Autodesk Fusion 360 part; units mm, degrees
note: some values were not read from the file. Set by a fixed rule: which sketch regions a step uses.
(part 11 of 15)
  line L8809 (248.7, -65.336) -> (248.925, -65.5074)
  line L8810 (248.339, -68.8671) -> (248.069, -68.9523)
  line L8811 (-57.7847, -68.2576) -> (-57.7166, -67.9835)
  line L8812 (-50.3027, -70.2857) -> (-50.4682, -70.3693)
  line L8813 (-55.7831, -66.6017) -> (-55.5017, -66.6261)
  line L8814 (249.602, -67.0076) -> (249.598, -67.1332)
  line L8815 (-57.536, -69.6196) -> (-57.6623, -69.3669)
  line L8816 (248.925, -65.5074) -> (249.123, -65.7087)
  line L8817 (-50.4436, -68.6079) -> (-50.2805, -68.696)
  line L8818 (-51.192, -70.3542) -> (-51.3539, -70.2637)
  line L8819 (249.598, -67.1332) -> (249.561, -67.4132)
  line L8820 (248.069, -68.9523) -> (247.791, -68.9987)
  line L8821 (-49.8621, -69.5102) -> (-49.8853, -69.6941)
  line L8822 (-55.0783, -70.4611) -> (-55.3476, -70.5462)
  line L8823 (249.291, -65.9359) -> (249.425, -66.1846)
  line L8824 (249.582, -66.7258) -> (249.602, -67.0076)
  line L8825 (-53.8561, -69.0071) -> (-53.9328, -69.279)
  line L8826 (-51.7461, -69.6551) -> (-51.7616, -69.4704)
  line L8827 (-51.4951, -70.1436) -> (-51.6102, -69.9983)
  line L8828 (-50.0204, -68.9579) -> (-49.9334, -69.1216)
  line L8829 (-51.6849, -69.1094) -> (-51.5956, -68.9469)
  line L8830 (-50.6467, -70.4192) -> (-50.8316, -70.4334)
  line L8831 (-51.1676, -68.6028) -> (-50.9897, -68.5505)
  line L8832 (-51.0157, -70.4115) -> (-51.192, -70.3542)
  line L8833 (-56.1893, -70.5661) -> (-56.4624, -70.4937)
  line L8834 (-51.7409, -69.2861) -> (-51.6849, -69.1094)
  line L8835 (-51.695, -69.8334) -> (-51.7461, -69.6551)
  line L8836 (-51.3319, -68.6887) -> (-51.1676, -68.6028)
  line L8837 (246.452, -68.6439) -> (246.233, -68.4655)
  line L8838 (246.233, -68.4655) -> (246.041, -68.2581)
  line L8839 (-51.6102, -69.9983) -> (-51.695, -69.8334)
  line L8840 (-49.8798, -69.2991) -> (-49.8617, -69.4836)
  line L8841 (249.484, -67.6851) -> (249.37, -67.9434)
  line L8842 (-50.0354, -70.0312) -> (-50.1566, -70.1716)
  line L8843 (248.828, -68.5879) -> (248.593, -68.7448)
  line L8844 (249.123, -65.7087) -> (249.291, -65.9359)
  line L8845 (-50.2805, -68.696) -> (-50.1376, -68.8142)
  line L8846 (-54.047, -69.5374) -> (-54.1965, -69.7771)
  line L8847 (-50.1566, -70.1716) -> (-50.3027, -70.2857)
  line L8848 (-49.9438, -69.87) -> (-50.0354, -70.0312)
  line L8849 (-51.3539, -70.2637) -> (-51.4951, -70.1436)
  line L8850 (-49.9334, -69.1216) -> (-49.8798, -69.2991)
  line L8851 (-51.7616, -69.4704) -> (-51.7409, -69.2861)
  line L8852 (-51.5956, -68.9469) -> (-51.4764, -68.8049)
  line L8853 (-50.9897, -68.5505) -> (-50.8051, -68.5337)
  line L8854 (249.039, -68.3994) -> (248.828, -68.5879)
  line L8855 (-50.6207, -68.553) -> (-50.4436, -68.6079)
  line L8856 (-50.4682, -70.3693) -> (-50.6467, -70.4192)
  line L8857 (-53.9328, -69.279) -> (-54.047, -69.5374)
  line L8858 (-57.8024, -68.821) -> (-57.8135, -68.5387)
  line L8859 (-49.8617, -69.4836) -> (-49.8621, -69.5102)
  line L8860 (-57.3754, -69.852) -> (-57.536, -69.6196)
  line L8861 (-57.8135, -68.5387) -> (-57.7847, -68.2576)
  line L8862 (-57.7517, -69.0989) -> (-57.8024, -68.821)
  line L8863 (-55.9087, -70.5993) -> (-56.1893, -70.5661)
  line L8864 (-57.4687, -67.4773) -> (-57.2938, -67.2555)
  line L8865 (-54.3783, -69.9933) -> (-54.5887, -70.1818)
  line L8866 (-50.8316, -70.4334) -> (-51.0157, -70.4115)
  line L8867 (-51.4764, -68.8049) -> (-51.3319, -68.6887)
  line L8868 (-50.1376, -68.8142) -> (-50.0204, -68.9579)
  line L8869 (-55.6263, -70.5926) -> (-55.9087, -70.5993)
  line L8870 (-56.0652, -66.6173) -> (-55.7831, -66.6017)
  line L8871 (-49.8853, -69.6941) -> (-49.9438, -69.87)
  line L8872 (88.5197, -67.9034) -> (88.3702, -68.1431)
  line L8873 (88.7322, -66.6857) -> (88.7522, -66.9675)
  line L8874 (246.328, -65.4666) -> (246.557, -65.3023)
  line L8875 (245.7, -66.3896) -> (245.806, -66.1277)
  line L8876 (247.634, -65.0078) -> (247.915, -65.0322)
  line L8877 (245.614, -67.2271) -> (245.603, -66.9448)
  line L8878 (86.3774, -68.9321) -> (86.1043, -68.8597)
  line L8879 (84.7819, -66.6237) -> (84.85, -66.3495)
  line L8880 (85.9579, -65.132) -> (86.2244, -65.0384)
  line L8881 (248.593, -68.7448) -> (248.339, -68.8671)
  line L8882 (245.603, -66.9448) -> (245.632, -66.6637)
  line L8883 (85.4773, -65.4265) -> (85.7072, -65.2622)
  line L8884 (243.131, -67.1021) -> (243.274, -67.2203)
  line L8885 (249.425, -66.1846) -> (249.523, -66.4496)
  line L8886 (86.6579, -68.9653) -> (86.3774, -68.9321)
  line L8887 (85.3831, -68.4255) -> (85.1913, -68.218)
  line L8888 (87.3402, -65.0559) -> (87.6037, -65.1579)
  line L8889 (87.8502, -65.2959) -> (88.0748, -65.4673)
  line L8890 (-50.8051, -68.5337) -> (-50.6207, -68.553)
  line L8891 (246.955, -68.8998) -> (246.694, -68.7896)
  line L8892 (87.065, -64.9921) -> (87.3402, -65.0559)
  line L8893 (245.806, -66.1277) -> (245.948, -65.8834)
  line L8894 (247.791, -68.9987) -> (247.508, -69.0054)
  line L8895 (88.7482, -67.0931) -> (88.7106, -67.3731)
  line L8896 (248.19, -65.096) -> (248.454, -65.1979)
  line L8897 (88.4408, -65.8959) -> (88.575, -66.1445)
  line L8898 (88.7522, -66.9675) -> (88.7482, -67.0931)
  line L8899 (247.352, -65.0234) -> (247.634, -65.0078)
  line L8900 (87.6037, -65.1579) -> (87.8502, -65.2959)
  line L8901 (88.273, -65.6686) -> (88.4408, -65.8959)
  line L8902 (88.3702, -68.1431) -> (88.1884, -68.3593)
  line L8903 (246.041, -68.2581) -> (245.881, -68.0257)
  line L8904 (247.915, -65.0322) -> (248.19, -65.096)
  line L8905 (245.632, -66.6637) -> (245.7, -66.3896)
  line L8906 (248.454, -65.1979) -> (248.7, -65.336)
  line L8907 (84.7531, -66.9047) -> (84.7819, -66.6237)
  line L8908 (84.85, -66.3495) -> (84.9561, -66.0876)
  line L8909 (88.6727, -66.4095) -> (88.7322, -66.6857)
  line L8910 (86.2244, -65.0384) -> (86.5015, -64.9833)
  line L8911 (246.808, -65.1721) -> (247.075, -65.0785)
  line L8912 (249.523, -66.4496) -> (249.582, -66.7258)
  line L8913 (88.7106, -67.3731) -> (88.6339, -67.645)
  line L8914 (88.0748, -65.4673) -> (88.273, -65.6686)
  line L8915 (247.228, -68.9722) -> (246.955, -68.8998)
  line L8916 (249.22, -68.1832) -> (249.039, -68.3994)
  line L8917 (245.665, -67.505) -> (245.614, -67.2271)
  line L8918 (246.557, -65.3023) -> (246.808, -65.1721)
  line L8919 (249.561, -67.4132) -> (249.484, -67.6851)
  line L8920 (246.694, -68.7896) -> (246.452, -68.6439)
  line L8921 (88.1884, -68.3593) -> (87.978, -68.5478)
  line L8922 (88.575, -66.1445) -> (88.6727, -66.4095)
  line L8923 (86.9404, -68.9586) -> (86.6579, -68.9653)
  line L8924 (245.755, -67.773) -> (245.665, -67.505)
  line L8925 (84.9044, -67.7329) -> (84.815, -67.4649)
  line L8926 (86.7836, -64.9678) -> (87.065, -64.9921)
  line L8927 (242.791, -66.9591) -> (242.968, -67.0139)
  line L8928 (246.123, -65.6616) -> (246.328, -65.4666)
  line L8929 (85.8442, -68.7495) -> (85.6021, -68.6038)
  line L8930 (85.1913, -68.218) -> (85.0307, -67.9856)
  line L8931 (247.075, -65.0785) -> (247.352, -65.0234)
  line L8932 (247.508, -69.0054) -> (247.228, -68.9722)
  line L8933 (245.881, -68.0257) -> (245.755, -67.773)
  line L8934 (88.6339, -67.645) -> (88.5197, -67.9034)
  line L8935 (245.948, -65.8834) -> (246.123, -65.6616)
  line L8936 (243.549, -67.9162) -> (243.526, -68.1002)
  line L8937 (241.816, -67.353) -> (241.935, -67.211)
  line L8938 (243.255, -68.5777) -> (243.109, -68.6918)
  line L8939 (241.67, -67.6922) -> (241.726, -67.5155)
  line L8940 (86.1043, -68.8597) -> (85.8442, -68.7495)
  line L8941 (242.58, -68.8395) -> (242.396, -68.8176)
  line L8942 (87.978, -68.5478) -> (87.7431, -68.7048)
  line L8943 (84.815, -67.4649) -> (84.7642, -67.187)
  line L8944 (243.109, -68.6918) -> (242.943, -68.7754)
  line L8945 (241.665, -68.0612) -> (241.65, -67.8765)
  line L8946 (243.467, -68.2761) -> (243.376, -68.4373)
  line L8947 (87.7431, -68.7048) -> (87.4884, -68.8271)
  line L8948 (242.943, -68.7754) -> (242.764, -68.8253)
  line L8949 (242.422, -66.9565) -> (242.606, -66.9397)
  line L8950 (85.0307, -67.9856) -> (84.9044, -67.7329)
  line L8951 (91.946, -66.9191) -> (92.1231, -66.9739)
  line L8952 (243.526, -68.1002) -> (243.467, -68.2761)
  line L8953 (85.098, -65.8434) -> (85.2729, -65.6215)
  line L8954 (243.478, -67.5277) -> (243.531, -67.7052)
  line L8955 (86.5015, -64.9833) -> (86.7836, -64.9678)
  line L8956 (242.396, -68.8176) -> (242.219, -68.7603)
  line L8957 (242.057, -68.6698) -> (241.916, -68.5496)
  line L8958 (241.716, -68.2394) -> (241.665, -68.0612)
  line L8959 (242.079, -67.0948) -> (242.244, -67.0089)
  line L8960 (91.2348, -67.0547) -> (91.3991, -66.9688)
  line L8961 (243.274, -67.2203) -> (243.391, -67.364)
  line L8962 (-60.4492, -66.8436) -> (-60.2861, -66.9318)
  line L8963 (92.6869, -67.6651) -> (92.705, -67.8497)
  line L8964 (92.6814, -68.0601) -> (92.6228, -68.2361)
  line L8965 (243.376, -68.4373) -> (243.255, -68.5777)
  line L8966 (92.264, -68.6518) -> (92.0985, -68.7354)
  line L8967 (92.705, -67.8497) -> (92.7046, -67.8762)
  line L8968 (91.7351, -68.7994) -> (91.551, -68.7775)
  line L8969 (92.0985, -68.7354) -> (91.9199, -68.7852)
  line L8970 (90.8206, -68.0211) -> (90.8051, -67.8364)
  line L8971 (92.7046, -67.8762) -> (92.6814, -68.0601)
  line L8972 (243.55, -67.8897) -> (243.549, -67.9162)
  line L8973 (241.65, -67.8765) -> (241.67, -67.6922)
  line L8974 (91.577, -66.9165) -> (91.7616, -66.8997)
  line L8975 (242.764, -68.8253) -> (242.58, -68.8395)
  line L8976 (242.606, -66.9397) -> (242.791, -66.9591)
  line L8977 (92.4101, -68.5376) -> (92.264, -68.6518)
  line L8978 (242.244, -67.0089) -> (242.422, -66.9565)
  line L8979 (241.726, -67.5155) -> (241.816, -67.353)
  line L8980 (91.2128, -68.6297) -> (91.0716, -68.5096)
  line L8981 (91.0716, -68.5096) -> (90.9564, -68.3643)
  line L8982 (85.2729, -65.6215) -> (85.4773, -65.4265)
  line L8983 (243.391, -67.364) -> (243.478, -67.5277)
  line L8984 (87.4884, -68.8271) -> (87.219, -68.9123)
  line L8985 (241.916, -68.5496) -> (241.801, -68.4043)
  line L8986 (243.531, -67.7052) -> (243.55, -67.8897)
  line L8987 (91.551, -68.7775) -> (91.3746, -68.7202)
  line L8988 (241.801, -68.4043) -> (241.716, -68.2394)
  line L8989 (84.7642, -67.187) -> (84.7531, -66.9047)
  line L8990 (241.935, -67.211) -> (242.079, -67.0948)
  line L8991 (92.2862, -67.0621) -> (92.4291, -67.1803)
  line L8992 (90.8717, -68.1994) -> (90.8206, -68.0211)
  line L8993 (242.219, -68.7603) -> (242.057, -68.6698)
  line L8994 (92.1231, -66.9739) -> (92.2862, -67.0621)
  line L8995 (87.219, -68.9123) -> (86.9404, -68.9586)
  line L8996 (85.6021, -68.6038) -> (85.3831, -68.4255)
  line L8997 (242.968, -67.0139) -> (243.131, -67.1021)
  line L8998 (84.9561, -66.0876) -> (85.098, -65.8434)
  line L8999 (85.7072, -65.2622) -> (85.9579, -65.132)
  line L9000 (-60.0261, -67.1936) -> (-59.939, -67.3574)
  line L9001 (-60.1433, -67.05) -> (-60.0261, -67.1936)
  line L9002 (-59.891, -67.9298) -> (-59.9495, -68.1058)
  line L9003 (-61.1732, -66.8385) -> (-60.9954, -66.7862)
  line L9004 (-60.6524, -68.6549) -> (-60.8372, -68.6692)
  line L9005 (-59.939, -67.3574) -> (-59.8854, -67.5348)
  line L9006 (-60.8372, -68.6692) -> (-61.0213, -68.6472)
  line L9007 (-60.1622, -68.4073) -> (-60.3083, -68.5215)
  line L9008 (-61.3595, -68.4995) -> (-61.5007, -68.3793)
  line L9009 (-60.8107, -66.7694) -> (-60.6263, -66.7888)
  line L9010 (-61.7673, -67.7061) -> (-61.7466, -67.5219)
  line L9011 (176.49, -67.4428) -> (176.44, -67.6091)
  line L9012 (90.9711, -67.3129) -> (91.0903, -67.1709)
  line L9013 (-61.0213, -68.6472) -> (-61.1977, -68.5899)
  line L9014 (-61.1977, -68.5899) -> (-61.3595, -68.4995)
  line L9015 (175.752, -66.56) -> (175.845, -66.5658)
  line L9016 (174.659, -68.0542) -> (174.491, -68.013)
  line L9017 (-60.2861, -66.9318) -> (-60.1433, -67.05)
  line L9018 (176.501, -67.2694) -> (176.49, -67.4428)
  line L9019 (92.5463, -67.3239) -> (92.6333, -67.4876)
  line L9020 (-60.9954, -66.7862) -> (-60.8107, -66.7694)
  line L9021 (-61.7466, -67.5219) -> (-61.6905, -67.3451)
  line L9022 (174.003, -67.3506) -> (174.014, -67.1772)
  line L9023 (91.9199, -68.7852) -> (91.7351, -68.7994)
  line L9024 (-61.6012, -67.1827) -> (-61.482, -67.0406)
  line L9025 (-59.9495, -68.1058) -> (-60.0411, -68.267)
  line L9026 (-61.3375, -66.9244) -> (-61.1732, -66.8385)
  line L9027 (176.471, -67.0982) -> (176.501, -67.2694)
  line L9028 (176.233, -67.8854) -> (176.088, -67.9806)
  line L9029 (-60.6263, -66.7888) -> (-60.4492, -66.8436)
  line L9030 (-61.5007, -68.3793) -> (-61.6159, -68.234)
  line L9031 (90.8051, -67.8364) -> (90.8257, -67.6521)
  line L9032 (-60.3083, -68.5215) -> (-60.4738, -68.6051)
  line L9033 (90.8818, -67.4754) -> (90.9711, -67.3129)
  line L9034 (-61.6159, -68.234) -> (-61.7006, -68.0691)
  line L9035 (174.151, -66.8607) -> (174.271, -66.7346)
  line L9036 (176.088, -67.9806) -> (175.925, -68.0399)
  line L9037 (175.845, -66.5658) -> (176.013, -66.607)
  line L9038 (92.5313, -68.3973) -> (92.4101, -68.5376)
  line L9039 (91.3991, -66.9688) -> (91.577, -66.9165)
  line L9040 (-61.6905, -67.3451) -> (-61.6012, -67.1827)
  line L9041 (-60.4738, -68.6051) -> (-60.6524, -68.6549)
  line L9042 (-59.8677, -67.7459) -> (-59.891, -67.9298)
  line L9043 (159.928, -66.686) -> (160.061, -66.7985)
  line L9044 (174.491, -68.013) -> (174.336, -67.934)
  line L9045 (174.579, -66.5801) -> (174.752, -66.56)
  line L9046 (174.014, -67.1772) -> (174.064, -67.0109)
  line L9047 (174.271, -66.7346) -> (174.416, -66.6394)
  line L9048 (176.168, -66.686) -> (176.301, -66.7985)
  line L9049 (-59.8854, -67.5348) -> (-59.8673, -67.7194)
  line L9050 (-61.7517, -67.8909) -> (-61.7673, -67.7061)
  line L9051 (174.101, -67.6816) -> (174.033, -67.5218)
  line L9052 (91.7616, -66.8997) -> (91.946, -66.9191)
  line L9053 (90.9564, -68.3643) -> (90.8717, -68.1994)
  line L9054 (92.4291, -67.1803) -> (92.5463, -67.3239)
  line L9055 (90.8257, -67.6521) -> (90.8818, -67.4754)
  line L9056 (91.0903, -67.1709) -> (91.2348, -67.0547)
  line L9057 (92.6228, -68.2361) -> (92.5313, -68.3973)
  line L9058 (-61.482, -67.0406) -> (-61.3375, -66.9244)
  line L9059 (-61.7006, -68.0691) -> (-61.7517, -67.8909)
  line L9060 (92.6333, -67.4876) -> (92.6869, -67.6651)
  line L9061 (-60.0411, -68.267) -> (-60.1622, -68.4073)
  line L9062 (91.3746, -68.7202) -> (91.2128, -68.6297)
  line L9063 (-59.8673, -67.7194) -> (-59.8677, -67.7459)
  line L9064 (158.339, -66.5801) -> (158.512, -66.56)
  line L9065 (268.083, -64.4506) -> (268.281, -64.652)
  line L9066 (159.512, -68.06) -> (158.512, -68.06)
  line L9067 (160.061, -66.7985) -> (160.163, -66.9384)
  line L9068 (267.611, -64.1412) -> (267.858, -64.2792)
  line L9069 (174.064, -67.0109) -> (174.151, -66.8607)
  line L9070 (268.76, -65.9509) -> (268.756, -66.0764)
  line L9071 (268.583, -65.1278) -> (268.68, -65.3929)
  line L9072 (268.281, -64.652) -> (268.449, -64.8792)
  line L9073 (268.68, -65.3929) -> (268.74, -65.6691)
  line L9074 (267.348, -64.0393) -> (267.611, -64.1412)
  line L9075 (264.772, -66.1703) -> (264.761, -65.888)
  line L9076 (264.858, -65.3328) -> (264.964, -65.071)
  line L9077 (176.013, -66.607) -> (176.168, -66.686)
  line L9078 (267.751, -67.6881) -> (267.496, -67.8104)
  line L9079 (264.964, -65.071) -> (265.106, -64.8267)
  line L9080 (159.993, -67.8854) -> (159.848, -67.9806)
  line L9081 (157.911, -66.8607) -> (158.031, -66.7346)
  line L9082 (174.752, -68.06) -> (174.659, -68.0542)
  line L9083 (176.403, -66.9384) -> (176.471, -67.0982)
  line L9084 (267.073, -63.9755) -> (267.348, -64.0393)
  line L9085 (160.261, -67.2694) -> (160.25, -67.4428)
  line L9086 (174.416, -66.6394) -> (174.579, -66.5801)
  line L9087 (159.685, -68.0399) -> (159.512, -68.06)
  line L9088 (174.752, -66.56) -> (175.752, -66.56)
  line L9089 (267.858, -64.2792) -> (268.083, -64.4506)
  line L9090 (160.231, -67.0982) -> (160.261, -67.2694)
  line L9091 (158.419, -68.0542) -> (158.251, -68.013)
  line L9092 (160.25, -67.4428) -> (160.2, -67.6091)
  line L9093 (160.113, -67.7593) -> (159.993, -67.8854)
  line L9094 (158.031, -66.7346) -> (158.176, -66.6394)
  line L9095 (176.353, -67.7593) -> (176.233, -67.8854)
  line L9096 (174.033, -67.5218) -> (174.003, -67.3506)
  line L9097 (158.176, -66.6394) -> (158.339, -66.5801)
  line L9098 (174.203, -67.8215) -> (174.101, -67.6816)
  line L9099 (267.227, -67.8956) -> (266.948, -67.942)
  line L9100 (266.112, -67.843) -> (265.852, -67.7329)
  line L9101 (157.861, -67.6816) -> (157.793, -67.5218)
  line L9102 (266.948, -67.942) -> (266.666, -67.9486)
  line L9103 (157.793, -67.5218) -> (157.763, -67.3506)
  line L9104 (159.605, -66.5658) -> (159.773, -66.607)
  line L9105 (158.512, -66.56) -> (159.512, -66.56)
  line L9106 (159.512, -66.56) -> (159.605, -66.5658)
  line L9107 (176.301, -66.7985) -> (176.403, -66.9384)
  line L9108 (159.773, -66.607) -> (159.928, -66.686)
  line L9109 (158.251, -68.013) -> (158.096, -67.934)
  line L9110 (157.774, -67.1772) -> (157.824, -67.0109)
  line L9111 (176.44, -67.6091) -> (176.353, -67.7593)
  line L9112 (174.336, -67.934) -> (174.203, -67.8215)
  line L9113 (160.163, -66.9384) -> (160.231, -67.0982)
  line L9114 (157.963, -67.8215) -> (157.861, -67.6816)
  line L9115 (268.378, -67.1264) -> (268.196, -67.3427)
  line L9116 (159.848, -67.9806) -> (159.685, -68.0399)
  line L9117 (268.642, -66.6283) -> (268.527, -66.8867)
  line L9118 (265.852, -67.7329) -> (265.61, -67.5872)
  line L9119 (265.61, -67.5872) -> (265.391, -67.4088)
  line L9120 (160.2, -67.6091) -> (160.113, -67.7593)
  line L9121 (158.512, -68.06) -> (158.419, -68.0542)
  line L9122 (268.718, -66.3564) -> (268.642, -66.6283)
  line L9123 (157.824, -67.0109) -> (157.911, -66.8607)
  line L9124 (175.925, -68.0399) -> (175.752, -68.06)
  line L9125 (175.752, -68.06) -> (174.752, -68.06)
  line L9126 (157.763, -67.3506) -> (157.774, -67.1772)
  line L9127 (158.096, -67.934) -> (157.963, -67.8215)
  line L9128 (67.7828, -67.9019) -> (67.5004, -67.9086)
  line L9129 (69.1154, -64.6119) -> (69.2833, -64.8391)
  line L9130 (67.2198, -67.8754) -> (66.9468, -67.803)
  line L9131 (261.948, -65.9024) -> (262.125, -65.9572)
  line L9132 (264.823, -66.4482) -> (264.772, -66.1703)
  line L9133 (266.791, -63.9511) -> (267.073, -63.9755)
  line L9134 (69.4174, -65.0878) -> (69.5152, -65.3528)
  line L9135 (267.986, -67.5312) -> (267.751, -67.6881)
  line L9136 (66.6866, -67.6928) -> (66.4446, -67.5471)
  line L9137 (266.666, -67.9486) -> (266.385, -67.9154)
  line L9138 (266.509, -63.9666) -> (266.791, -63.9511)
  line L9139 (265.966, -64.1153) -> (266.232, -64.0217)
  line L9140 (262.125, -65.9572) -> (262.288, -66.0454)
  line L9141 (67.0669, -63.9817) -> (67.3439, -63.9266)
  line L9142 (265.281, -64.6048) -> (265.485, -64.4098)
  line L9143 (262.288, -66.0454) -> (262.431, -66.1636)
  line L9144 (66.4446, -67.5471) -> (66.2255, -67.3687)
  line L9145 (69.5946, -65.9108) -> (69.5907, -66.0364)
  line L9146 (68.9172, -64.4106) -> (69.1154, -64.6119)
  line L9147 (69.0309, -67.3026) -> (68.8204, -67.4911)
  line L9148 (68.4462, -64.1011) -> (68.6927, -64.2392)
  line L9149 (69.5907, -66.0364) -> (69.5531, -66.3164)
  line L9150 (68.0615, -67.8555) -> (67.7828, -67.9019)
  line L9151 (69.5152, -65.3528) -> (69.5747, -65.629)
  line L9152 (69.4764, -66.5883) -> (69.3621, -66.8467)
  line L9153 (264.912, -66.7162) -> (264.823, -66.4482)
  line L9154 (68.8204, -67.4911) -> (68.5855, -67.6481)
  line L9155 (265.485, -64.4098) -> (265.715, -64.2456)
  line L9156 (268.756, -66.0764) -> (268.718, -66.3564)
  line L9157 (268.449, -64.8792) -> (268.583, -65.1278)
  line L9158 (69.2126, -67.0864) -> (69.0309, -67.3026)
  line L9159 (65.7986, -65.0309) -> (65.9404, -64.7866)
  line L9160 (65.6244, -65.5669) -> (65.6925, -65.2928)
  line L9161 (65.8731, -66.9289) -> (65.7468, -66.6762)
  line L9162 (262.707, -66.8595) -> (262.683, -67.0435)
  line L9163 (262.683, -67.0435) -> (262.625, -67.2194)
  line L9164 (265.715, -64.2456) -> (265.966, -64.1153)
  line L9165 (264.761, -65.888) -> (264.79, -65.607)
  line L9166 (265.199, -67.2013) -> (265.038, -66.9689)
  line L9167 (264.79, -65.607) -> (264.858, -65.3328)
  line L9168 (265.391, -67.4088) -> (265.199, -67.2013)
  line L9169 (68.3309, -67.7703) -> (68.0615, -67.8555)
  line L9170 (69.5531, -66.3164) -> (69.4764, -66.5883)
  line L9171 (66.0337, -67.1613) -> (65.8731, -66.9289)
  line L9172 (267.496, -67.8104) -> (267.227, -67.8956)
  line L9173 (268.74, -65.6691) -> (268.76, -65.9509)
  line L9174 (268.527, -66.8867) -> (268.378, -67.1264)
  line L9175 (268.196, -67.3427) -> (267.986, -67.5312)
  line L9176 (69.5747, -65.629) -> (69.5946, -65.9108)
  line L9177 (68.5855, -67.6481) -> (68.3309, -67.7703)
  line L9178 (265.106, -64.8267) -> (265.281, -64.6048)
  line L9179 (67.5004, -67.9086) -> (67.2198, -67.8754)
  line L9180 (68.1827, -63.9992) -> (68.4462, -64.1011)
  line L9181 (68.6927, -64.2392) -> (68.9172, -64.4106)
  line L9182 (65.5956, -65.848) -> (65.6244, -65.5669)
  line L9183 (67.9075, -63.9354) -> (68.1827, -63.9992)
  line L9184 (66.3198, -64.3698) -> (66.5496, -64.2055)
  line L9185 (65.6574, -66.4082) -> (65.6067, -66.1303)
  line L9186 (265.038, -66.9689) -> (264.912, -66.7162)
  line L9187 (69.2833, -64.8391) -> (69.4174, -65.0878)
  line L9188 (66.8003, -64.0753) -> (67.0669, -63.9817)
  line L9189 (266.232, -64.0217) -> (266.509, -63.9666)
  line L9190 (69.3621, -66.8467) -> (69.2126, -67.0864)
  line L9191 (266.385, -67.9154) -> (266.112, -67.843)
  line L9192 (72.941, -67.6786) -> (72.7624, -67.7285)
  line L9193 (71.7243, -66.4187) -> (71.8136, -66.2562)
  line L9194 (72.9656, -65.9172) -> (73.1287, -66.0053)
  line L9195 (261.377, -67.7035) -> (261.215, -67.6131)
  line L9196 (262.707, -66.833) -> (262.707, -66.8595)
  line L9197 (73.3887, -66.2672) -> (73.4758, -66.4309)
  line L9198 (262.635, -66.471) -> (262.689, -66.6485)
  line L9199 (261.764, -65.883) -> (261.948, -65.9024)
  line L9200 (261.092, -66.1542) -> (261.237, -66.0381)
  line L9201 (71.7989, -67.3075) -> (71.7141, -67.1426)
  line L9202 (286.857, -63.5848) -> (287.104, -63.7228)
  line L9203 (73.5293, -66.6084) -> (73.5474, -66.7929)
  line L9204 (287.104, -63.7228) -> (287.328, -63.8942)
  line L9205 (287.526, -64.0955) -> (287.694, -64.3228)
  line L9206 (262.548, -66.3073) -> (262.635, -66.471)
  line L9207 (261.579, -65.8998) -> (261.764, -65.883)
  line L9208 (72.2171, -67.6635) -> (72.0553, -67.573)
  line L9209 (65.6067, -66.1303) -> (65.5956, -65.848)
  line L9210 (262.689, -66.6485) -> (262.707, -66.833)
  line L9211 (67.626, -63.911) -> (67.9075, -63.9354)
  line L9212 (73.5474, -66.7929) -> (73.5471, -66.8195)
  line L9213 (262.412, -67.521) -> (262.266, -67.6351)
  line L9214 (73.5238, -67.0034) -> (73.4653, -67.1793)
  line L9215 (65.7468, -66.6762) -> (65.6574, -66.4082)
  line L9216 (260.884, -66.4587) -> (260.973, -66.2963)
  line L9217 (261.074, -67.4929) -> (260.959, -67.3476)
  line L9218 (260.828, -66.6355) -> (260.884, -66.4587)
  line L9219 (287.328, -63.8942) -> (287.526, -64.0955)
  line L9220 (260.973, -66.2963) -> (261.092, -66.1542)
  line L9221 (71.9141, -67.4528) -> (71.7989, -67.3075)
  line L9222 (66.5496, -64.2055) -> (66.8003, -64.0753)
  line L9223 (261.737, -67.7828) -> (261.553, -67.7608)
  line L9224 (260.959, -67.3476) -> (260.874, -67.1827)
  line L9225 (261.237, -66.0381) -> (261.401, -65.9522)
  line L9226 (72.0772, -65.998) -> (72.2416, -65.9121)
  line L9227 (287.694, -64.3228) -> (287.828, -64.5714)
  line L9228 (262.431, -66.1636) -> (262.548, -66.3073)
  line L9229 (286.319, -63.419) -> (286.594, -63.4828)
  line L9230 (262.533, -67.3806) -> (262.412, -67.521)
  line L9231 (73.3737, -67.3405) -> (73.2526, -67.4809)
  line L9232 (71.7141, -67.1426) -> (71.663, -66.9644)
  line L9233 (260.823, -67.0045) -> (260.807, -66.8197)
  line L9234 (262.625, -67.2194) -> (262.533, -67.3806)
  line L9235 (67.3439, -63.9266) -> (67.626, -63.911)
  line L9236 (65.9404, -64.7866) -> (66.1153, -64.5648)
  line L9237 (261.553, -67.7608) -> (261.377, -67.7035)
  line L9238 (73.2715, -66.1235) -> (73.3887, -66.2672)
  line L9239 (261.922, -67.7686) -> (261.737, -67.7828)
  line L9240 (72.7885, -65.8623) -> (72.9656, -65.9172)
  line L9241 (73.1287, -66.0053) -> (73.2715, -66.1235)
  line L9242 (261.215, -67.6131) -> (261.074, -67.4929)
  line L9243 (260.874, -67.1827) -> (260.823, -67.0045)
  line L9244 (261.401, -65.9522) -> (261.579, -65.8998)
  line L9245 (66.1153, -64.5648) -> (66.3198, -64.3698)
  line L9246 (262.266, -67.6351) -> (262.101, -67.7187)
  line L9247 (73.1065, -67.595) -> (72.941, -67.6786)
  line L9248 (260.807, -66.8197) -> (260.828, -66.6355)
  line L9249 (72.6041, -65.8429) -> (72.7885, -65.8623)
  line L9250 (66.9468, -67.803) -> (66.6866, -67.6928)
  line L9251 (73.5471, -66.8195) -> (73.5238, -67.0034)
  line L9252 (73.4758, -66.4309) -> (73.5293, -66.6084)
  line L9253 (66.2255, -67.3687) -> (66.0337, -67.1613)
  line L9254 (262.101, -67.7187) -> (261.922, -67.7686)
  line L9255 (65.6925, -65.2928) -> (65.7986, -65.0309)
  line L9256 (287.624, -66.57) -> (287.442, -66.7862)
  line L9257 (48.2546, -67.3521) -> (47.9741, -67.3189)
  line L9258 (284.018, -65.6139) -> (284.007, -65.3316)
  line L9259 (284.104, -64.7764) -> (284.21, -64.5145)
  line L9260 (47.701, -67.2465) -> (47.4409, -67.1364)
  line L9261 (49.4469, -63.6827) -> (49.6715, -63.8541)
  line L9262 (49.3398, -67.0916) -> (49.0851, -67.2139)
  line L9263 (50.1717, -64.5313) -> (50.2694, -64.7964)
  line L9264 (47.4409, -67.1364) -> (47.1988, -66.9906)
  line L9265 (287.828, -64.5714) -> (287.926, -64.8364)
  line L9266 (286.997, -67.1317) -> (286.742, -67.254)
  line L9267 (284.351, -64.2702) -> (284.526, -64.0484)
  line L9268 (285.098, -67.1764) -> (284.856, -67.0307)
  line L9269 (284.961, -63.6891) -> (285.211, -63.5589)
  line L9270 (50.3449, -65.4799) -> (50.3073, -65.7599)
  line L9271 (47.1988, -66.9906) -> (46.9798, -66.8123)
  line L9272 (285.478, -63.4653) -> (285.755, -63.4102)
  line L9273 (72.2416, -65.9121) -> (72.4194, -65.8598)
  line L9274 (286.194, -67.3855) -> (285.911, -67.3922)
  line L9275 (285.631, -67.359) -> (285.358, -67.2866)
  line L9276 (73.4653, -67.1793) -> (73.3737, -67.3405)
  line L9277 (72.7624, -67.7285) -> (72.5775, -67.7427)
  line L9278 (287.231, -66.9747) -> (286.997, -67.1317)
  line L9279 (287.986, -65.1126) -> (288.006, -65.3944)
  line L9280 (287.964, -65.8) -> (287.887, -66.0719)
  line L9281 (71.9328, -66.1142) -> (72.0772, -65.998)
  line L9282 (287.442, -66.7862) -> (287.231, -66.9747)
  line L9283 (284.445, -66.6449) -> (284.284, -66.4125)
  line L9284 (286.594, -63.4828) -> (286.857, -63.5848)
  line L9285 (286.742, -67.254) -> (286.473, -67.3392)
  line L9286 (284.526, -64.0484) -> (284.731, -63.8534)
  line L9287 (284.284, -66.4125) -> (284.158, -66.1598)
  line L9288 (285.358, -67.2866) -> (285.098, -67.1764)
  line L9289 (288.006, -65.3944) -> (288.002, -65.52)
  line L9290 (288.002, -65.52) -> (287.964, -65.8)
  line L9291 (287.773, -66.3303) -> (287.624, -66.57)
  line L9292 (284.856, -67.0307) -> (284.637, -66.8524)
  line L9293 (72.0553, -67.573) -> (71.9141, -67.4528)
  line L9294 (284.158, -66.1598) -> (284.068, -65.8918)
  line L9295 (287.926, -64.8364) -> (287.986, -65.1126)
  line L9296 (72.5775, -67.7427) -> (72.3934, -67.7208)
  line L9297 (286.473, -67.3392) -> (286.194, -67.3855)
  line L9298 (50.3289, -65.0725) -> (50.3488, -65.3543)
  line L9299 (287.887, -66.0719) -> (287.773, -66.3303)
  line L9300 (72.4194, -65.8598) -> (72.6041, -65.8429)
  line L9301 (71.663, -66.9644) -> (71.6475, -66.7797)
  line L9302 (73.2526, -67.4809) -> (73.1065, -67.595)
  line L9303 (284.21, -64.5145) -> (284.351, -64.2702)
  line L9304 (49.7851, -66.7462) -> (49.5747, -66.9347)
  line L9305 (48.6617, -63.379) -> (48.9369, -63.4428)
  line L9306 (71.8136, -66.2562) -> (71.9328, -66.1142)
  line L9307 (71.6475, -66.7797) -> (71.6682, -66.5954)
  line L9308 (284.007, -65.3316) -> (284.035, -65.0506)
  line L9309 (284.035, -65.0506) -> (284.104, -64.7764)
  line L9310 (50.3488, -65.3543) -> (50.3449, -65.4799)
  line L9311 (284.637, -66.8524) -> (284.445, -66.6449)
  line L9312 (49.9669, -66.5299) -> (49.7851, -66.7462)
  line L9313 (49.2004, -63.5447) -> (49.4469, -63.6827)
  line L9314 (48.5371, -67.3455) -> (48.2546, -67.3521)
  line L9315 (285.911, -67.3922) -> (285.631, -67.359)
  line L9316 (284.068, -65.8918) -> (284.018, -65.6139)
  line L9317 (72.3934, -67.7208) -> (72.2171, -67.6635)
  line L9318 (284.731, -63.8534) -> (284.961, -63.6891)
  line L9319 (71.6682, -66.5954) -> (71.7243, -66.4187)
  line L9320 (46.788, -66.6048) -> (46.6274, -66.3724)
  line L9321 (285.755, -63.4102) -> (286.037, -63.3947)
  line L9322 (48.3803, -63.3546) -> (48.6617, -63.379)
  line L9323 (281.953, -66.2765) -> (281.952, -66.3031)
  line L9324 (47.3039, -63.6491) -> (47.5546, -63.5188)
  line L9325 (281.929, -66.487) -> (281.871, -66.6629)
  line L9326 (46.3498, -65.2915) -> (46.3786, -65.0105)
  line L9327 (281.677, -65.6071) -> (281.794, -65.7508)
  line L9328 (281.346, -67.1623) -> (281.168, -67.2121)
  line L9329 (281.371, -65.4008) -> (281.534, -65.489)
  line L9330 (49.8697, -64.0555) -> (50.0375, -64.2827)
  line L9331 (281.935, -66.092) -> (281.953, -66.2765)
  line L9332 (46.5011, -66.1197) -> (46.4117, -65.8517)
  line L9333 (281.881, -65.9145) -> (281.935, -66.092)
  line L9334 (46.6947, -64.2302) -> (46.8696, -64.0083)
  line L9335 (281.952, -66.3031) -> (281.929, -66.487)
  line L9336 (49.5747, -66.9347) -> (49.3398, -67.0916)
  line L9337 (47.074, -63.8133) -> (47.3039, -63.6491)
  line L9338 (54.2781, -66.447) -> (54.2195, -66.6229)
  line L9339 (46.5528, -64.4745) -> (46.6947, -64.2302)
  line L9340 (280.338, -65.5978) -> (280.483, -65.4816)
  line L9341 (50.2694, -64.7964) -> (50.3289, -65.0725)
  line L9342 (281.871, -66.6629) -> (281.779, -66.8242)
  line L9343 (281.009, -65.3266) -> (281.194, -65.346)
  line L9344 (46.9798, -66.8123) -> (46.788, -66.6048)
  line L9345 (48.8157, -67.2991) -> (48.5371, -67.3455)
  line L9346 (46.3609, -65.5738) -> (46.3498, -65.2915)
  line L9347 (280.799, -67.2044) -> (280.623, -67.1471)
  line L9348 (46.6274, -66.3724) -> (46.5011, -66.1197)
  line L9349 (50.3073, -65.7599) -> (50.2306, -66.0318)
  line L9350 (54.1429, -65.7108) -> (54.23, -65.8745)
  line L9351 (286.037, -63.3947) -> (286.319, -63.419)
  line L9352 (280.483, -65.4816) -> (280.647, -65.3957)
  line L9353 (54.0068, -66.9244) -> (53.8607, -67.0386)
  line L9354 (53.5427, -65.3059) -> (53.7198, -65.3607)
  line L9355 (46.4117, -65.8517) -> (46.3609, -65.5738)
  line L9356 (47.8211, -63.4252) -> (48.0982, -63.3701)
  line L9357 (281.512, -67.0787) -> (281.346, -67.1623)
  line L9358 (281.658, -66.9645) -> (281.512, -67.0787)
  line L9359 (48.9369, -63.4428) -> (49.2004, -63.5447)
  line L9360 (48.0982, -63.3701) -> (48.3803, -63.3546)
  line L9361 (281.779, -66.8242) -> (281.658, -66.9645)
  line L9362 (54.2195, -66.6229) -> (54.128, -66.7841)
  line L9363 (280.623, -67.1471) -> (280.461, -67.0566)
  line L9364 (46.4467, -64.7363) -> (46.5528, -64.4745)
  line L9365 (281.194, -65.346) -> (281.371, -65.4008)
  line L9366 (50.1164, -66.2902) -> (49.9669, -66.5299)
  line L9367 (49.0851, -67.2139) -> (48.8157, -67.2991)
  line L9368 (46.3786, -65.0105) -> (46.4467, -64.7363)
  line L9369 (54.3013, -66.263) -> (54.2781, -66.447)
  line L9370 (53.8607, -67.0386) -> (53.6952, -67.1222)
  line L9371 (53.8829, -65.4489) -> (54.0258, -65.5671)
  line L9372 (280.983, -67.2263) -> (280.799, -67.2044)
  line L9373 (46.8696, -64.0083) -> (47.074, -63.8133)
  line L9374 (280.053, -66.2633) -> (280.074, -66.079)
  line L9375 (54.128, -66.7841) -> (54.0068, -66.9244)
  line L9376 (285.211, -63.5589) -> (285.478, -63.4653)
  line L9377 (47.5546, -63.5188) -> (47.8211, -63.4252)
  line L9378 (281.534, -65.489) -> (281.677, -65.6071)
  line L9379 (47.9741, -67.3189) -> (47.701, -67.2465)
  line L9380 (50.2306, -66.0318) -> (50.1164, -66.2902)
  line L9381 (281.794, -65.7508) -> (281.881, -65.9145)
  line L9382 (50.0375, -64.2827) -> (50.1717, -64.5313)
  line L9383 (49.6715, -63.8541) -> (49.8697, -64.0555)
  line L9384 (213.502, -58.2989) -> (213.52, -58.4834)
  line L9385 (252.973, -65.2497) -> (253.136, -65.3379)
  line L9386 (212.028, -59.2635) -> (211.887, -59.1433)
  line L9387 (280.319, -66.9365) -> (280.204, -66.7912)
  line L9388 (53.1737, -65.3033) -> (53.3583, -65.2865)
  line L9389 (52.5531, -66.7511) -> (52.4684, -66.5862)
  line L9390 (211.62, -58.4701) -> (211.641, -58.2859)
  line L9391 (211.697, -58.1092) -> (211.786, -57.9467)
  line L9392 (213.101, -57.6958) -> (213.244, -57.814)
  line L9393 (280.068, -66.448) -> (280.053, -66.2633)
  line L9394 (280.219, -65.7398) -> (280.338, -65.5978)
  line L9395 (213.496, -58.6939) -> (213.438, -58.8698)
  line L9396 (212.05, -57.6885) -> (212.214, -57.6026)
  line L9397 (53.1477, -67.1643) -> (52.9713, -67.107)
  line L9398 (212.214, -57.6026) -> (212.392, -57.5502)
  line L9399 (211.887, -59.1433) -> (211.771, -58.998)
  line L9400 (253.136, -65.3379) -> (253.279, -65.456)
  line L9401 (52.4684, -66.5862) -> (52.4173, -66.408)
  line L9402 (54.23, -65.8745) -> (54.2836, -66.052)
  line L9403 (280.204, -66.7912) -> (280.12, -66.6263)
  line L9404 (280.13, -65.9023) -> (280.219, -65.7398)
  line L9405 (253.279, -65.456) -> (253.396, -65.5997)
  line L9406 (54.2836, -66.052) -> (54.3017, -66.2365)
  line L9407 (253.396, -65.5997) -> (253.483, -65.7634)
  line L9408 (54.0258, -65.5671) -> (54.1429, -65.7108)
  line L9409 (54.3017, -66.2365) -> (54.3013, -66.263)
  line L9410 (53.3318, -67.1863) -> (53.1477, -67.1643)
  line L9411 (52.9713, -67.107) -> (52.8095, -67.0166)
  line L9412 (52.6683, -66.8964) -> (52.5531, -66.7511)
  line L9413 (52.8315, -65.4416) -> (52.9958, -65.3557)
  line L9414 (52.9958, -65.3557) -> (53.1737, -65.3033)
  line L9415 (280.461, -67.0566) -> (280.319, -66.9365)
  line L9416 (280.647, -65.3957) -> (280.825, -65.3434)
  line L9417 (213.079, -59.2855) -> (212.913, -59.3691)
  line L9418 (280.12, -66.6263) -> (280.068, -66.448)
  line L9419 (213.346, -59.031) -> (213.225, -59.1714)
  line L9420 (211.786, -57.9467) -> (211.905, -57.8047)
  line L9421 (52.4785, -65.8622) -> (52.5678, -65.6998)
  line L9422 (212.735, -59.419) -> (212.55, -59.4332)
  line L9423 (52.5678, -65.6998) -> (52.687, -65.5577)
  line L9424 (280.825, -65.3434) -> (281.009, -65.3266)
  line L9425 (53.6952, -67.1222) -> (53.5166, -67.172)
  line L9426 (52.4173, -66.408) -> (52.4018, -66.2232)
  line L9427 (280.074, -66.079) -> (280.13, -65.9023)
  line L9428 (52.4018, -66.2232) -> (52.4224, -66.039)
  line L9429 (213.225, -59.1714) -> (213.079, -59.2855)
  line L9430 (213.52, -58.5099) -> (213.496, -58.6939)
  line L9431 (281.168, -67.2121) -> (280.983, -67.2263)
  line L9432 (52.8095, -67.0166) -> (52.6683, -66.8964)
  line L9433 (52.687, -65.5577) -> (52.8315, -65.4416)
  line L9434 (253.483, -65.7634) -> (253.537, -65.9409)
  line L9435 (213.244, -57.814) -> (213.361, -57.9577)
  line L9436 (252.796, -65.1949) -> (252.973, -65.2497)
  line L9437 (212.392, -57.5502) -> (212.577, -57.5334)
  line L9438 (212.913, -59.3691) -> (212.735, -59.419)
  line L9439 (213.438, -58.8698) -> (213.346, -59.031)
  line L9440 (213.448, -58.1214) -> (213.502, -58.2989)
  line L9441 (211.641, -58.2859) -> (211.697, -58.1092)
  line L9442 (211.905, -57.8047) -> (212.05, -57.6885)
  line L9443 (53.5166, -67.172) -> (53.3318, -67.1863)
  line L9444 (52.4224, -66.039) -> (52.4785, -65.8622)
  line L9445 (53.7198, -65.3607) -> (53.8829, -65.4489)
  line L9446 (253.537, -65.9409) -> (253.555, -66.1255)
  line L9447 (53.3583, -65.2865) -> (53.5427, -65.3059)
  line L9448 (81.2072, -66.8655) -> (81.066, -66.7453)
  line L9449 (80.9508, -66.6) -> (80.866, -66.4351)
  line L9450 (272.131, -64.193) -> (272.294, -64.2811)
  line L9451 (271.098, -64.39) -> (271.243, -64.2738)
  line L9452 (82.6812, -65.9009) -> (82.6993, -66.0854)
  line L9453 (211.771, -58.998) -> (211.687, -58.8331)
  line L9454 (212.938, -57.6076) -> (213.101, -57.6958)
  line L9455 (82.5256, -66.633) -> (82.4045, -66.7733)
  line L9456 (213.361, -57.9577) -> (213.448, -58.1214)
  line L9457 (81.066, -66.7453) -> (80.9508, -66.6)
  line L9458 (81.5453, -67.0132) -> (81.369, -66.9559)
  line L9459 (271.559, -65.9966) -> (271.382, -65.9393)
  line L9460 (270.828, -65.2402) -> (270.813, -65.0555)
  line L9461 (271.407, -64.1879) -> (271.585, -64.1356)
  line L9462 (271.079, -65.7287) -> (270.964, -65.5833)
  line L9463 (62.9599, -64.1529) -> (63.123, -64.2411)
  line L9464 (63.2659, -64.3593) -> (63.3831, -64.5029)
  line L9465 (80.8201, -65.8879) -> (80.8762, -65.7111)
  line L9466 (271.769, -64.1187) -> (271.954, -64.1381)
  line L9467 (62.7828, -64.0981) -> (62.9599, -64.1529)
  line L9468 (80.8762, -65.7111) -> (80.9655, -65.5487)
  line L9469 (81.9143, -67.021) -> (81.7294, -67.0352)
  line L9470 (82.6993, -66.0854) -> (82.699, -66.1119)
  line L9471 (271.243, -64.2738) -> (271.407, -64.1879)
  line L9472 (272.641, -64.7067) -> (272.695, -64.8842)
  line L9473 (81.369, -66.9559) -> (81.2072, -66.8655)
  line L9474 (272.539, -65.6163) -> (272.418, -65.7567)
  line L9475 (272.418, -65.7567) -> (272.272, -65.8708)
  line L9476 (80.7994, -66.0721) -> (80.8201, -65.8879)
  line L9477 (82.6172, -66.4718) -> (82.5256, -66.633)
  line L9478 (81.2291, -65.2905) -> (81.3935, -65.2046)
  line L9479 (63.123, -64.2411) -> (63.2659, -64.3593)
  line L9480 (270.879, -65.4184) -> (270.828, -65.2402)
  line L9481 (272.106, -65.9544) -> (271.928, -66.0043)
  line L9482 (271.221, -65.8488) -> (271.079, -65.7287)
  line L9483 (272.631, -65.4551) -> (272.539, -65.6163)
  line L9484 (272.689, -65.2792) -> (272.631, -65.4551)
  line L9485 (212.761, -57.5528) -> (212.938, -57.6076)
  line L9486 (212.366, -59.4112) -> (212.19, -59.3539)
  line L9487 (211.636, -58.6549) -> (211.62, -58.4701)
  line L9488 (82.699, -66.1119) -> (82.6757, -66.2959)
  line L9489 (81.3935, -65.2046) -> (81.5713, -65.1522)
  line L9490 (81.756, -65.1354) -> (81.9404, -65.1548)
  line L9491 (272.294, -64.2811) -> (272.437, -64.3993)
  line L9492 (82.2584, -66.8875) -> (82.0929, -66.9711)
  line L9493 (80.9655, -65.5487) -> (81.0847, -65.4066)
  line L9494 (213.52, -58.4834) -> (213.52, -58.5099)
  line L9495 (81.0847, -65.4066) -> (81.2291, -65.2905)
  line L9496 (81.7294, -67.0352) -> (81.5453, -67.0132)
  line L9497 (271.954, -64.1381) -> (272.131, -64.193)
  line L9498 (82.0929, -66.9711) -> (81.9143, -67.021)
  line L9499 (272.554, -64.543) -> (272.641, -64.7067)
  line L9500 (82.4045, -66.7733) -> (82.2584, -66.8875)
  line L9501 (212.55, -59.4332) -> (212.366, -59.4112)
  line L9502 (270.813, -65.0555) -> (270.833, -64.8712)
  line L9503 (272.437, -64.3993) -> (272.554, -64.543)
  line L9504 (272.272, -65.8708) -> (272.106, -65.9544)
  line L9505 (271.585, -64.1356) -> (271.769, -64.1187)
  line L9506 (80.8149, -66.2569) -> (80.7994, -66.0721)
  line L9507 (81.5713, -65.1522) -> (81.756, -65.1354)
  line L9508 (211.687, -58.8331) -> (211.636, -58.6549)
  line L9509 (212.19, -59.3539) -> (212.028, -59.2635)
  line L9510 (82.6757, -66.2959) -> (82.6172, -66.4718)
  line L9511 (80.866, -66.4351) -> (80.8149, -66.2569)
  line L9512 (62.9353, -65.9144) -> (62.7568, -65.9642)
  line L9513 (271.743, -66.0185) -> (271.559, -65.9966)
  line L9514 (61.6574, -65.2002) -> (61.6419, -65.0154)
  line L9515 (176.013, -64.067) -> (176.168, -64.146)
  line L9516 (63.4701, -64.6666) -> (63.5237, -64.8441)
  line L9517 (62.0716, -64.2337) -> (62.2359, -64.1478)
  line L9518 (61.9271, -64.3499) -> (62.0716, -64.2337)
  line L9519 (174.003, -64.8106) -> (174.014, -64.6372)
  line L9520 (174.203, -65.2815) -> (174.101, -65.1416)
  line L9521 (63.3681, -65.5763) -> (63.2469, -65.7166)
  line L9522 (272.695, -64.8842) -> (272.713, -65.0687)
  line L9523 (63.3831, -64.5029) -> (63.4701, -64.6666)
  line L9524 (63.2469, -65.7166) -> (63.1008, -65.8308)
  line L9525 (176.471, -64.5582) -> (176.501, -64.7294)
  line L9526 (271.382, -65.9393) -> (271.221, -65.8488)
  line L9527 (272.712, -65.0953) -> (272.689, -65.2792)
  line L9528 (174.752, -64.02) -> (175.752, -64.02)
  line L9529 (61.6625, -64.8311) -> (61.7186, -64.6544)
  line L9530 (62.3878, -65.9565) -> (62.2115, -65.8992)
  line L9531 (63.4597, -65.4151) -> (63.3681, -65.5763)
  line L9532 (62.0496, -65.8088) -> (61.9084, -65.6886)
  line L9533 (176.49, -64.9028) -> (176.44, -65.0691)
  line L9534 (174.064, -64.4709) -> (174.151, -64.3207)
  line L9535 (63.1008, -65.8308) -> (62.9353, -65.9144)
  line L9536 (62.2115, -65.8992) -> (62.0496, -65.8088)
  line L9537 (174.101, -65.1416) -> (174.033, -64.9818)
  line L9538 (176.301, -64.2585) -> (176.403, -64.3984)
  line L9539 (174.416, -64.0994) -> (174.579, -64.0401)
  line L9540 (159.773, -64.067) -> (159.928, -64.146)
  line L9541 (174.014, -64.6372) -> (174.064, -64.4709)
  line L9542 (174.271, -64.1946) -> (174.416, -64.0994)
  line L9543 (61.9084, -65.6886) -> (61.7932, -65.5433)
  line L9544 (176.168, -64.146) -> (176.301, -64.2585)
  line L9545 (61.7186, -64.6544) -> (61.8079, -64.4919)
  line L9546 (61.6419, -65.0154) -> (61.6625, -64.8311)
  line L9547 (159.928, -64.146) -> (160.061, -64.2585)
  line L9548 (62.5719, -65.9785) -> (62.3878, -65.9565)
  line L9549 (61.7932, -65.5433) -> (61.7085, -65.3784)
  line L9550 (174.752, -65.52) -> (174.659, -65.5142)
  line L9551 (62.2359, -64.1478) -> (62.4138, -64.0955)
  line L9552 (63.5182, -65.2391) -> (63.4597, -65.4151)
  line L9553 (174.579, -64.0401) -> (174.752, -64.02)
  line L9554 (62.7568, -65.9642) -> (62.5719, -65.9785)
  line L9555 (62.5984, -64.0787) -> (62.7828, -64.0981)
  line L9556 (175.752, -65.52) -> (174.752, -65.52)
  line L9557 (63.5418, -65.0287) -> (63.5414, -65.0552)
  line L9558 (270.833, -64.8712) -> (270.89, -64.6945)
  line L9559 (271.928, -66.0043) -> (271.743, -66.0185)
  line L9560 (61.8079, -64.4919) -> (61.9271, -64.3499)
  line L9561 (61.7085, -65.3784) -> (61.6574, -65.2002)
  line L9562 (63.5414, -65.0552) -> (63.5182, -65.2391)
  line L9563 (176.44, -65.0691) -> (176.353, -65.2193)
  line L9564 (174.151, -64.3207) -> (174.271, -64.1946)
  line L9565 (62.4138, -64.0955) -> (62.5984, -64.0787)
  line L9566 (270.979, -64.532) -> (271.098, -64.39)
  line L9567 (175.752, -64.02) -> (175.845, -64.0258)
  line L9568 (176.403, -64.3984) -> (176.471, -64.5582)
  line L9569 (176.501, -64.7294) -> (176.49, -64.9028)
  line L9570 (272.713, -65.0687) -> (272.712, -65.0953)
  line L9571 (63.5237, -64.8441) -> (63.5418, -65.0287)
  line L9572 (174.033, -64.9818) -> (174.003, -64.8106)
  line L9573 (175.845, -64.0258) -> (176.013, -64.067)
  line L9574 (270.89, -64.6945) -> (270.979, -64.532)
  line L9575 (270.964, -65.5833) -> (270.879, -65.4184)
  line L9576 (158.339, -64.0401) -> (158.512, -64.02)
  line L9577 (160.061, -64.2585) -> (160.163, -64.3984)
  line L9578 (291.377, -63.6365) -> (291.54, -63.7247)
  line L9579 (158.419, -65.5142) -> (158.251, -65.473)
  line L9580 (157.793, -64.9818) -> (157.763, -64.8106)
  line L9581 (157.774, -64.6372) -> (157.824, -64.4709)
  line L9582 (159.993, -65.3454) -> (159.848, -65.4406)
  line L9583 (157.763, -64.8106) -> (157.774, -64.6372)
  line L9584 (291.887, -64.1503) -> (291.94, -64.3278)
  line L9585 (160.2, -65.0691) -> (160.113, -65.2193)
  line L9586 (159.512, -65.52) -> (158.512, -65.52)
  line L9587 (159.685, -65.4999) -> (159.512, -65.52)
  line L9588 (157.911, -64.3207) -> (158.031, -64.1946)
  line L9589 (291.2, -63.5817) -> (291.377, -63.6365)
  line L9590 (290.325, -65.1722) -> (290.21, -65.0269)
  line L9591 (43.8773, -63.6846) -> (44.0201, -63.8028)
  line L9592 (176.353, -65.2193) -> (176.233, -65.3454)
  line L9593 (160.261, -64.7294) -> (160.25, -64.9028)
  line L9594 (290.21, -65.0269) -> (290.125, -64.862)
  line L9595 (158.096, -65.394) -> (157.963, -65.2815)
  line L9596 (290.074, -64.6838) -> (290.059, -64.499)
  line L9597 (174.659, -65.5142) -> (174.491, -65.473)
  line L9598 (291.8, -63.9866) -> (291.887, -64.1503)
  line L9599 (290.059, -64.499) -> (290.079, -64.3148)
  line L9600 (291.935, -64.7228) -> (291.876, -64.8987)
  line L9601 (158.512, -65.52) -> (158.419, -65.5142)
  line L9602 (291.785, -65.0599) -> (291.664, -65.2002)
  line L9603 (44.0201, -63.8028) -> (44.1373, -63.9465)
  line L9604 (160.25, -64.9028) -> (160.2, -65.0691)
  line L9605 (160.163, -64.3984) -> (160.231, -64.5582)
  line L9606 (291.173, -65.4478) -> (290.989, -65.4621)
  line L9607 (174.336, -65.394) -> (174.203, -65.2815)
  line L9608 (44.1373, -63.9465) -> (44.2243, -64.1102)
  line L9609 (291.352, -65.398) -> (291.173, -65.4478)
  line L9610 (290.225, -63.9756) -> (290.344, -63.8335)
  line L9611 (159.848, -65.4406) -> (159.685, -65.4999)
  line L9612 (291.683, -63.8429) -> (291.8, -63.9866)
  line L9613 (291.54, -63.7247) -> (291.683, -63.8429)
  line L9614 (160.113, -65.2193) -> (159.993, -65.3454)
  line L9615 (158.031, -64.1946) -> (158.176, -64.0994)
  line L9616 (290.804, -65.4401) -> (290.628, -65.3828)
  line L9617 (290.628, -65.3828) -> (290.466, -65.2924)
  line L9618 (291.876, -64.8987) -> (291.785, -65.0599)
  line L9619 (291.958, -64.5388) -> (291.935, -64.7228)
  line L9620 (158.512, -64.02) -> (159.512, -64.02)
  line L9621 (157.824, -64.4709) -> (157.911, -64.3207)
  line L9622 (175.925, -65.4999) -> (175.752, -65.52)
  line L9623 (174.491, -65.473) -> (174.336, -65.394)
  line L9624 (291.94, -64.3278) -> (291.958, -64.5123)
  line L9625 (290.079, -64.3148) -> (290.135, -64.138)
  line L9626 (44.2243, -64.1102) -> (44.2779, -64.2877)
  line L9627 (290.135, -64.138) -> (290.225, -63.9756)
  line L9628 (291.015, -63.5623) -> (291.2, -63.5817)
  line L9629 (158.176, -64.0994) -> (158.339, -64.0401)
  line L9630 (290.83, -63.5791) -> (291.015, -63.5623)
  line L9631 (290.125, -64.862) -> (290.074, -64.6838)
  line L9632 (159.605, -64.0258) -> (159.773, -64.067)
  line L9633 (157.963, -65.2815) -> (157.861, -65.1416)
  line L9634 (157.861, -65.1416) -> (157.793, -64.9818)
  line L9635 (176.088, -65.4406) -> (175.925, -65.4999)
  line L9636 (158.251, -65.473) -> (158.096, -65.394)
  line L9637 (159.512, -64.02) -> (159.605, -64.0258)
  line L9638 (160.231, -64.5582) -> (160.261, -64.7294)
  line L9639 (176.233, -65.3454) -> (176.088, -65.4406)
  line L9640 (42.8038, -65.2523) -> (42.6627, -65.1321)
  line L9641 (42.6627, -65.1321) -> (42.5475, -64.9868)
  line L9642 (42.4627, -64.8219) -> (42.4116, -64.6437)
  line L9643 (187.899, -64.4555) -> (187.656, -64.3098)
  line L9644 (187.437, -64.1315) -> (187.246, -63.924)
  line L9645 (190.688, -63.351) -> (190.574, -63.6094)
  line L9646 (291.958, -64.5123) -> (291.958, -64.5388)
  line L9647 (187.085, -63.6916) -> (186.959, -63.4389)
  line L9648 (190.727, -62.1155) -> (190.787, -62.3917)
  line L9649 (186.869, -63.1709) -> (186.819, -62.893)
  line L9650 (42.4116, -64.6437) -> (42.3961, -64.459)
  line L9651 (190.327, -61.3746) -> (190.495, -61.6019)
  line L9652 (42.8258, -63.6773) -> (42.9901, -63.5914)
  line L9653 (190.425, -63.8491) -> (190.243, -64.0654)
  line L9654 (188.712, -64.6713) -> (188.432, -64.6381)
  line L9655 (186.819, -62.893) -> (186.807, -62.6107)
  line L9656 (186.959, -63.4389) -> (186.869, -63.1709)
  line L9657 (290.989, -65.4621) -> (290.804, -65.4401)
  line L9658 (43.168, -63.539) -> (43.3527, -63.5222)
  line L9659 (291.664, -65.2002) -> (291.518, -65.3144)
  line L9660 (42.5622, -63.9355) -> (42.6813, -63.7935)
  line L9661 (188.995, -64.6647) -> (188.712, -64.6713)
  line L9662 (190.803, -62.7991) -> (190.765, -63.0791)
  line L9663 (290.466, -65.2924) -> (290.325, -65.1722)
  line L9664 (42.5475, -64.9868) -> (42.4627, -64.8219)
  line L9665 (44.0012, -65.1602) -> (43.8551, -65.2743)
  line L9666 (43.3527, -63.5222) -> (43.5371, -63.5416)
  line L9667 (190.243, -64.0654) -> (190.032, -64.2538)
  line L9668 (190.765, -63.0791) -> (190.688, -63.351)
  line L9669 (189.119, -60.6982) -> (189.395, -60.7619)
  line L9670 (189.658, -60.8639) -> (189.905, -61.0019)
  line L9671 (43.142, -65.4001) -> (42.9657, -65.3428)
  line L9672 (43.8551, -65.2743) -> (43.6896, -65.3579)
  line L9673 (189.905, -61.0019) -> (190.129, -61.1733)
  line L9674 (187.656, -64.3098) -> (187.437, -64.1315)
  line L9675 (186.836, -62.3297) -> (186.904, -62.0555)
  line L9676 (290.344, -63.8335) -> (290.488, -63.7174)
  line L9677 (44.2779, -64.2877) -> (44.296, -64.4722)
  line L9678 (42.9657, -65.3428) -> (42.8038, -65.2523)
  line L9679 (291.518, -65.3144) -> (291.352, -65.398)
  line L9680 (44.2957, -64.4987) -> (44.2724, -64.6827)
  line L9681 (190.129, -61.1733) -> (190.327, -61.3746)
  line L9682 (43.7142, -63.5964) -> (43.8773, -63.6846)
  line L9683 (190.787, -62.3917) -> (190.807, -62.6735)
  line L9684 (190.574, -63.6094) -> (190.425, -63.8491)
  line L9685 (43.6896, -65.3579) -> (43.511, -65.4078)
  line L9686 (186.807, -62.6107) -> (186.836, -62.3297)
  line L9687 (190.629, -61.8505) -> (190.727, -62.1155)
  line L9688 (44.2139, -64.8586) -> (44.1223, -65.0198)
  line L9689 (187.246, -63.924) -> (187.085, -63.6916)
  line L9690 (44.1223, -65.0198) -> (44.0012, -65.1602)
  line L9691 (44.2724, -64.6827) -> (44.2139, -64.8586)
  line L9692 (43.3261, -65.422) -> (43.142, -65.4001)
  line L9693 (189.395, -60.7619) -> (189.658, -60.8639)
  line L9694 (42.4728, -64.098) -> (42.5622, -63.9355)
  line L9695 (42.3961, -64.459) -> (42.4168, -64.2747)
  line L9696 (42.6813, -63.7935) -> (42.8258, -63.6773)
  line L9697 (43.511, -65.4078) -> (43.3261, -65.422)
  line L9698 (290.488, -63.7174) -> (290.653, -63.6315)
  line L9699 (44.296, -64.4722) -> (44.2957, -64.4987)
  line L9700 (42.9901, -63.5914) -> (43.168, -63.539)
  line L9701 (43.5371, -63.5416) -> (43.7142, -63.5964)
  line L9702 (290.653, -63.6315) -> (290.83, -63.5791)